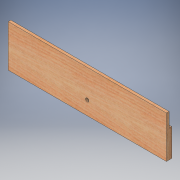
# Autodesk Inventor part: SkinnySideWOpposite
Saved by Autodesk Inventor 2016 (Build 200138000, 138)
## iProperties
Created: 2016-02-11
Part Number: SkinnySideWOpposite
Material: Wood (Birch)
Document SubType Name: Modeling
Designer: ron
Density: 0.55 g/cm^3
Appearance: Birch - Natural Polished
Mass: 823.974 g
Surface Area: 2104.06 cm^2
Volume: 1498.13 cm^3
Author: ron
Autodesk Inventor part; units mm, degrees
ref_plane "YZ Plane" through (0, 0, 0) normal (1, 0, 0) x (0, 1, 0)
ref_plane "XZ Plane" through (0, 0, 0) normal (0, 1, 0) x (-1, 0, 0)
sketch "Sketch1" plane through (0, 0, 0) normal (1, 0, 0) x (0, 1, 0)
  line L0 (0, 0) -> (155.1, 0)
  line L1 (155.1, 0) -> (155.1, -10)
  line L2 (0, -20) -> (0, 0)
  line L3 (155.1, -10) -> (101.6, -10)
  line L4 (101.6, -10) -> (101.6, -20)
  line L5 (101.6, -20) -> (0, -20)
  dimension "d0" = 53.5
  dimension "d1" = 155.1
  dimension "d2" = 10
  dimension "d3" = 10
  dimension "d4" = 20
  constraints: 12 end point, 3 horizontal, 2 parallel, 1 perpendicular
  measures "d0" distance of L1.end L3.end
  measures "d1" distance between parallel lines of L1 L2
  measures "d2" distance between parallel lines of L3 L5
  measures "d3" distance between parallel lines of L0 L3
  measures "d4" vertical distance of L4.end L0.end
extrude "Extrusion1" add sketch "Sketch1" along normal blind 584.6
ref_plane "Work Plane2" through (609.4222, 0, -20) normal (0, 0, -1) x (-1, 0, 0)
sketch "Sketch4" plane through (0, 0, 0) normal (0, 0, 1) x (1, 0, 0)
  line L0 (0, 0) -> (0, 155.1) projected
  line L1 (0, 0) -> (292.3032, 0)
  line L2 (0, 0) -> (584.6, 0) projected
  line L3 (292.3032, 50.8) -> (292.3032, 0)
  dimension "d38" = 292.3032
  dimension "d39" = 50.8
  constraints: 4 end point, 1 perpendicular, 1 point on line
  measures "d38" distance of L0.start L1.end
  measures "d39" distance of L3.start L1.end
hole "Hole1" at (292.3032, 50.8, 0) direction (0, 0, -1) diameter 12.7 end through all
body "Solid1"
